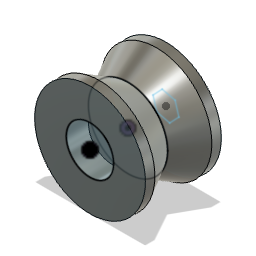
Spool v3 (Autodesk Fusion 360 design; units mm, degrees)
Autodesk Fusion 360 part; units mm, degrees
sketch "Sketch1" plane through (0, 0, 0) normal (0, 0, 1) x (1, 0, 0)
  circle A0 centre (0, 0) radius 17.5
  dimension "d1" = 35
  constraint coincident A0.centre origin
  measures "d1" diameter of A0
ref_plane "WorkPlane1" through (0, 0, 18) normal (0, 0, 1) x (1, 0, 0)
sketch "Sketch2" plane through (0, 0, 18) normal (0, 0, 1) x (1, 0, 0)
  circle A0 centre (0, 0) radius 17.5
  dimension "d3" = 35
  constraint coincident A0.centre origin
  measures "d3" diameter of A0
ref_plane "WorkPlane2" through (0, 0, 9) normal (0, 0, 1) x (1, 0, 0)
sketch "Sketch3" plane through (0, 0, 9) normal (0, 0, 1) x (1, 0, 0)
  circle A0 centre (0, 0) radius 12.5
  dimension "d5" = 25
  constraint coincident A0.centre origin
  measures "d5" diameter of A0
loft "Loft1" add profiles "Sketch2", "Sketch3" section 1 section 2
loft "Loft2" add profiles "Sketch1" section 1 section 2 face at (-3.3879, -0.621, 9)
extrude "Extrude1" add 1 faces at (4.4225, -5.9212, 18) along direction (0, 0, 1) blind 3
extrude "Extrude2" add 1 faces at (4.4225, -5.9212, 0) along direction (0, 0, -1) blind 3
sketch "Sketch4" plane through (0, 0, -3) normal (0, 0, -1) x (-1, 0, 0)
  circle A0 centre (0, 0) radius 17.5
  line L0 (2.8885, -3.049) -> (4.0848, 0.977)
  line L1 (4.0848, 0.977) -> (1.1962, 4.026)
  line L2 (1.1962, 4.026) -> (-2.8885, 3.049)
  line L3 (-2.8885, 3.049) -> (-4.0848, -0.977)
  line L4 (-4.0848, -0.977) -> (-1.1962, -4.026)
  line L5 (-1.1962, -4.026) -> (2.8885, -3.049)
  dimension "d10" = 4.2
  constraint coincident A0.centre origin
  measures "d10" distance of L0.start A0.centre
extrude "Extrude3" cut sketch "Sketch4" against normal blind 15 contours L0 L1 L2 L3 L4 L5
sketch "Sketch5" plane through (0, 0, 21) normal (0, 0, 1) x (1, 0, 0)
  circle A0 centre (0, 0) radius 17.5
sketch "Sketch6" plane through (0, 0, 21) normal (0, 0, 1) x (1, 0, 0)
  circle A0 centre (0, 0) radius 7.5
  dimension "d13" = 15
  constraint coincident A0.centre origin
  measures "d13" diameter of A0
extrude "Extrude4" cut sketch "Sketch6" against normal blind 7
sketch "Sketch7" plane through (0, 0, 21) normal (0, 0, 1) x (1, 0, 0)
  circle A0 centre (0, 0) radius 7.5
  dimension "d16" = 15
  constraint coincident A0.centre origin
  measures "d16" diameter of A0
sketch "Sketch8" plane through (0, 0, 21) normal (0, 0, 1) x (1, 0, 0)
  circle A0 centre (0, 0) radius 2.5
  dimension "d17" = 5
  constraint coincident A0.centre origin
  measures "d17" diameter of A0
extrude "Extrude5" cut sketch "Sketch8" against normal blind 9
equation "d4 = ( 18 / 2 ) * 1 mm"
